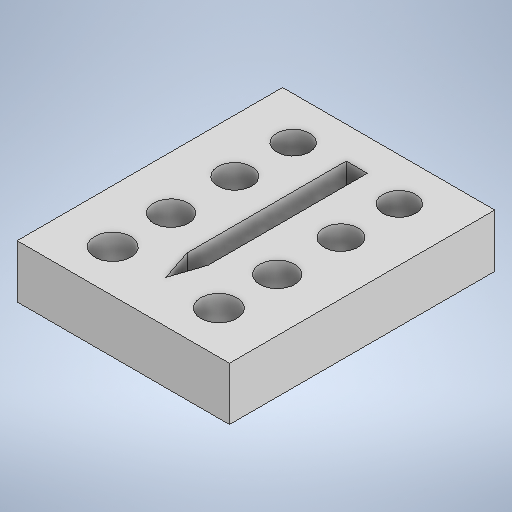
# Autodesk Inventor part: PAACF测试板
Saved by Autodesk Inventor 2025.2 (Build 292293000, 293)
## iProperties
Created: 2025-11-05
Part Number: PAACF测试板
Material: 常规
Document SubType Name: Modeling
Designer: BO‘S_SLAVE
Density: 1 g/cm^3
Appearance: 默认
Author: BO‘S_SLAVE
Autodesk Inventor part; units mm, degrees
ref_plane "YZ Plane" through (0, 0, 0) normal (1, 0, 0) x (0, 1, 0)
ref_plane "XZ Plane" through (0, 0, 0) normal (0, 1, 0) x (-1, 0, 0)
ref_plane "XY Plane" through (0, 0, 0) normal (0, 0, 1) x (1, 0, 0)
sketch "草图1" plane through (0, 0, 0) normal (0, 1, 0) x (-1, 0, 0)
  line L0 (0, 0) -> (-20, 0)
  line L1 (-20, 0) -> (-20, 25)
  line L2 (-20, 25) -> (0, 25)
  line L3 (0, 25) -> (0, 0)
  circle A0 centre (-5, 15.5) radius 1.65
  circle A1 centre (-5, 9.5) radius 1.6
  circle A2 centre (-5, 4) radius 1.55
  circle A3 centre (-5, 21) radius 1.7
  line L4 (0, 12.5) -> (-20, 12.5)
  line L5 (-10, 0) -> (-10, 25)
  circle A4 centre (-15, 15.5) radius 1.65
  circle A5 centre (-15, 9.5) radius 1.6
  circle A6 centre (-15, 4) radius 1.55
  circle A7 centre (-15, 21) radius 1.7
  line L6 (-11, 3) -> (-9, 3)
  line L7 (-9, 3) -> (-9, 18)
  line L8 (-9, 18) -> (-11, 18)
  line L9 (-11, 18) -> (-11, 3)
  line L10 (-11, 18) -> (-10, 21)
  line L11 (-9, 18) -> (-10, 21)
  dimension "d0" = 20
  dimension "d1" = 25
  dimension "d2" = 3.3
  dimension "d3" = 3.2
  dimension "d4" = 3.1
  dimension "d5" = 3.4
  dimension "d6" = 4
  dimension "d7" = 5
  dimension "d9" = 3
  dimension "d10" = 5
  dimension "d11" = 5
  dimension "d12" = 3
  dimension "d13" = 5
  dimension "d14" = 4
  dimension "d17" = 2
  dimension "d18" = 15
  dimension "d19" = 9
  dimension "d20" = 3
  dimension "d21" = 3
  constraints: 24 end point, 8 centre point, 4 midpoint, 4 parallel, 4 symmetric about line, 2 horizontal, 2 perpendicular, 1 point on line, 4 other
  measures "d0" distance between parallel lines of L3 L1
  measures "d1" distance between parallel lines of L2 L0
  measures "d2" diameter of A0
  measures "d3" diameter of A1
  measures "d4" diameter of A2
  measures "d5" diameter of A3
  measures "d6" distance from line of L0 A2.centre
  measures "d7" distance from line of L3 A2.centre
  measures "d9" distance from line of L4 A1.centre
  measures "d10" distance from line of L3 A1.centre
  measures "d11" distance from line of L3 A0.centre
  measures "d12" distance from line of L4 A0.centre
  measures "d13" distance from line of L3 A3.centre
  measures "d14" distance from line of L2 A3.centre
  measures "d17" distance between parallel lines of L7 L9
  measures "d18" distance between parallel lines of L8 L6
  measures "d19" distance between parallel lines of L1 L9
  measures "d20" distance between parallel lines of L0 L6
  measures "d21" distance from line of L8 L10.end
extrude "拉伸1" add sketch "草图1" along normal blind 5 contours L0 L5 L6 L7 L4 L3 | L0 L1 L4 L9 L6 L5 | L4 L7 L11 L5 L2 L3 | L1 L2 L5 L10 L9 L4
